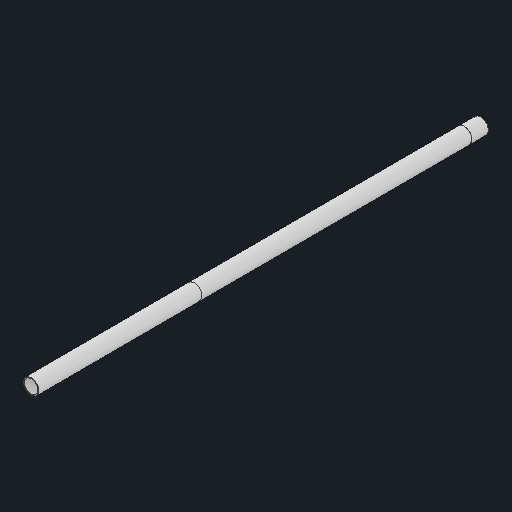
# Autodesk Inventor part: PIPE
Saved by Autodesk Inventor 2026.1 (Build 301233020, 233B)
## iProperties
Created: 2025-12-25
Part Number: PIPE
Material: Generic
Document SubType Name: Modeling
Designer: kngob
Density: 1 g/cm^3
Appearance: Default
Author: kngob
Autodesk Inventor part; units mm, degrees
ref_plane "YZ Plane" through (0, 0, 0) normal (1, 0, 0) x (0, 1, 0)
ref_plane "XZ Plane" through (0, 0, 0) normal (0, 1, 0) x (-1, 0, 0)
ref_plane "XY Plane" through (0, 0, 0) normal (0, 0, 1) x (1, 0, 0)
sketch "Sketch1" plane through (0, 0, 0) normal (0, 0, 1) x (1, 0, 0)
  circle A0 centre (0, 0) radius 9.25
  circle A1 centre (0, 0) radius 8.25
  dimension "d0" = 18.5
  dimension "d1" = 1
  constraints: 2 centre point, 1 coincident
  measures "d0" diameter of A0
  measures "d1" radial gap between concentric circles of A0 A1
extrude "Extrusion1" add sketch "Sketch1" along normal blind 200 and the other way blind 350
sketch "Sketch2" plane through (0, 0, 0) normal (1, 0, 0) x (0, 1, 0)
  line L0 (136.6486, 0) -> (-136.6486, 0)
  point P0 (0, 0)
  point P1 (0, 0)
  constraints: 2 end point, 1 coincident, 1 horizontal, 1 midpoint
bend part "Bend Part1" radius 60 angle 0.1 line through (0, 136.6486, 0) along (0, -1, 0) centre toward (1, 0, 0) moving side (0, 0, 1) both sides no
sketch "Sketch3" plane through (0, 0, 0) normal (1, 0, 0) x (0, 1, 0)
  line L0 (-36.06, -330) -> (87.8962, -330)
  line L1 (-9.25, -350) -> (9.25, -350) projected
  point P0 (0, 0)
  dimension "d8" = 20
  constraints: 2 end point, 1 horizontal
  measures "d8" distance between parallel lines of L1 L0
bend part "Bend Part2" radius 60 angle 0.1 line through (0, -36.06, -330) along (0, 1, 0) centre toward (1, 0, 0) moving side (0, 0, 1) both sides no
equation "\"d7\" = PIPEBEND1"
equation "\"d10\" = PIPEBEND2"
equation "\"PIPEBEND1\" = 0.1deg"
equation "\"PIPEBEND2\" = 0.1deg"
body "Solid1"
